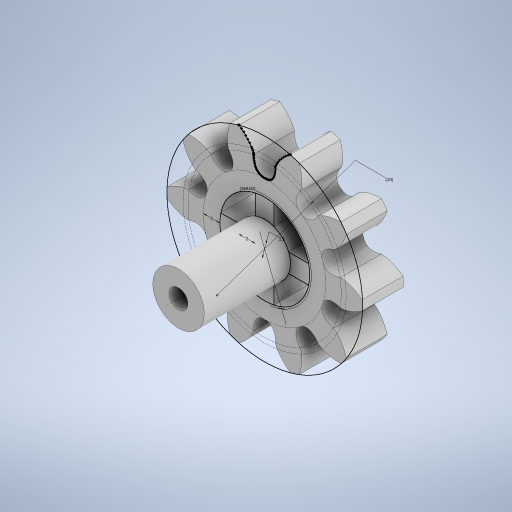
# Autodesk Inventor part: pinion_V3
Saved by Autodesk Inventor 2023 (Build 270158000, 158)
## iProperties
Created: 2022-11-24
Part Number: pinion_V3
Material: Generic
Document SubType Name: Modeling
Designer: shrey
Density: 1 g/cm^3
Appearance: Default
Author: shrey
Autodesk Inventor part; units mm, degrees
ref_plane "YZ Plane" through (0, 0, 0) normal (1, 0, 0) x (0, 1, 0)
ref_plane "XZ Plane" through (0, 0, 0) normal (0, 1, 0) x (-1, 0, 0)
ref_plane "XY Plane" through (0, 0, 0) normal (0, 0, 1) x (1, 0, 0)
sketch "Sketch1" plane through (0, 0, 0) normal (0, 0, 1) x (1, 0, 0)
  spline S0 degree 3 poles (-3.1449, 11.5806) (-3.0482, 11.5076) (-2.8549, 11.3615) (-2.5801, 11.1235) (-2.3181, 10.8715) (-2.0723, 10.6037) (-1.845, 10.3199) (-1.6746, 10.0692) (-1.5527, 9.8598) (-1.4703, 9.6979) (-1.3965, 9.5315) (-1.3613, 9.4156) (-1.3436, 9.3576) knots 0 0 0 0 0.125009 0.250018 0.375026 0.500029 0.625027 0.750014 0.81252 0.875024 0.937523 1 1 1 1
  spline S1 degree 3 poles (-1.3436, 9.3576) (-1.3456, 9.303) (-1.3494, 9.1938) (-1.3453, 9.0299) (-1.3323, 8.8664) (-1.3062, 8.7045) (-1.2743, 8.5436) (-1.2254, 8.3869) (-1.166, 8.2341) (-1.0913, 8.0878) (-1.0006, 7.951) (-0.8946, 7.8256) (-0.7725, 7.7154) (-0.6351, 7.6254) (-0.4861, 7.5557) (-0.3538, 7.5202) (-0.2459, 7.5023) (-0.1365, 7.4984) (0, 7.5011) (0.1365, 7.4984) (0.2459, 7.5023) (0.3538, 7.5202) (0.4861, 7.5557) (0.6351, 7.6254) (0.7725, 7.7154) (0.8946, 7.8256) (1.0006, 7.951) (1.0913, 8.0878) (1.166, 8.2341) (1.2254, 8.3869) (1.2743, 8.5436) (1.3062, 8.7045) (1.3323, 8.8664) (1.3453, 9.0299) (1.3494, 9.1938) (1.3456, 9.303) (1.3436, 9.3576) knots 0 0 0 0 0.016389 0.032777 0.049165 0.065552 0.081938 0.098325 0.114709 0.131097 0.147483 0.163864 0.180243 0.196616 0.21299 0.229355 0.237552 0.245745 0.262134 0.278522 0.286715 0.294912 0.311278 0.327651 0.344025 0.360403 0.376784 0.393171 0.409559 0.425942 0.44233 0.458716 0.475102 0.49149 0.507879 0.524268 0.524268 0.524268 0.524268
  spline S2 degree 3 poles (1.3436, 9.3576) (1.3613, 9.4156) (1.3965, 9.5315) (1.4703, 9.6979) (1.5527, 9.8598) (1.6746, 10.0692) (1.845, 10.3199) (2.0723, 10.6037) (2.3181, 10.8715) (2.5801, 11.1235) (2.8549, 11.3615) (3.0482, 11.5076) (3.1449, 11.5806) knots 0 0 0 0 0.062477 0.124976 0.18748 0.249986 0.374973 0.499971 0.624974 0.749982 0.874991 1 1 1 1
  circle A0 centre (0, 0) radius 7.5 construction
  circle A1 centre (0, 0) radius 9.3969 construction
  circle A2 centre (0, 0) radius 10 construction
  circle A3 centre (0, 0) radius 12
  circle A4 centre (0, 0) radius 1.15
  circle A5 centre (0, 0) radius 5.5
  circle A6 centre (0, 0) radius 3.15
  line L0 (-1.15, 2.9326) -> (-1.15, 5.3784)
  line L1 (1.15, 2.9326) -> (1.15, 5.3784)
  line L2 (-2.9326, -1.15) -> (-5.3784, -1.15)
  line L3 (-2.9326, 1.15) -> (-5.3784, 1.15)
  line L4 (1.15, -2.9326) -> (1.15, -5.3784)
  line L5 (-1.15, -2.9326) -> (-1.15, -5.3784)
  line L6 (2.9326, 1.15) -> (5.3784, 1.15)
  line L7 (2.9326, -1.15) -> (5.3784, -1.15)
  point P0 (-2.8575, 11.3584)
  point P1 (-2.5823, 11.1211)
  point P2 (-2.3208, 10.8689)
  point P3 (-2.0754, 10.601)
  point P4 (-1.8488, 10.317)
  point P5 (-1.6453, 10.0161)
  point P6 (-1.5542, 9.859)
  point P7 (-1.4717, 9.6971)
  point P8 (-1.4, 9.5302)
  point P9 (-1.3478, 9.1938)
  point P10 (-1.3438, 9.0299)
  point P11 (-1.3301, 8.8666)
  point P12 (-1.3053, 8.7047)
  point P13 (-1.2715, 8.5443)
  point P14 (-1.2237, 8.3876)
  point P15 (-1.1635, 8.2352)
  point P16 (-1.0887, 8.0894)
  point P17 (-0.998, 7.9529)
  point P18 (-0.8919, 7.8281)
  point P19 (-0.7699, 7.7188)
  point P20 (-0.6331, 7.6288)
  point P21 (-0.4845, 7.5602)
  point P22 (-0.3267, 7.5166)
  point P23 (-0.2457, 7.5041)
  point P24 (-0.1639, 7.4999)
  point P25 (0, 7.5)
  point P26 (0.1639, 7.4999)
  point P27 (0.2457, 7.5041)
  point P28 (0.3267, 7.5166)
  point P29 (0.4845, 7.5602)
  point P30 (0.6331, 7.6288)
  point P31 (0.7699, 7.7188)
  point P32 (0.8919, 7.8281)
  point P33 (0.998, 7.9529)
  point P34 (1.0887, 8.0894)
  point P35 (1.1635, 8.2352)
  point P36 (1.2237, 8.3876)
  point P37 (1.2715, 8.5443)
  point P38 (1.3053, 8.7047)
  point P39 (1.3301, 8.8666)
  point P40 (1.3438, 9.0299)
  point P41 (1.3478, 9.1938)
  point P42 (1.4, 9.5302)
  point P43 (1.4717, 9.6971)
  point P44 (1.5542, 9.859)
  point P45 (1.6453, 10.0161)
  point P46 (1.8488, 10.317)
  point P47 (2.0754, 10.601)
  point P48 (2.3208, 10.8689)
  point P49 (2.5823, 11.1211)
  point P50 (2.8575, 11.3584)
  point P51 (5.3784, -1.15)
  point P52 (2.9326, -1.15)
  point P53 (-1.15, -5.3784)
  point P54 (-2.9326, -1.15)
  point P55 (-5.3784, -1.15)
  point P56 (-5.3784, 1.15)
  point P57 (2.9326, 1.15)
  dimension "d2" = 2.3
  dimension "d3" = 2
  dimension "d4" = 2
  dimension "d7" = 360
  dimension "d18" = 20
  constraints: 16 end point, 7 centre point, 6 point on circle, 2 tangent, 1 coincident, 1 parallel, 1 vertical, 142 other
  measures "d2" diameter of A4
  measures "d3" radial gap between concentric circles of A0 A5
  measures "d4" radial gap between concentric circles of A4 A6
  measures "d18" diameter of A2
extrude "Extrusion1" add sketch "Sketch1" against normal blind 5 contours A3 S2 S1 S0 | S0 S1 S2 A3 | A4 | A5 L7 A6 L6 | L6 A6 L1 A5 | A5 L4 A6 L7 | L1 A6 L0 A5 | A6 | A5 L5 A6 L4 | L0 A6 L3 A5 | A5 L2 A6 L5 | L3 A6 L2 A5
extrude "Extrusion2" cut sketch "Sketch1" against normal through all contours A3 S2 S1 S0 picked at (0.367, 10.5472)
pattern_circular "Circular Pattern1" count 10 over 360 about axis through (0, 0, 0) along (0, 0, -1) of "Extrusion2"
extrude "Extrusion3" cut sketch "Sketch1" against normal through all contours A4 | L6 A6 L1 A5 | A5 L4 A6 L7 | L0 A6 L3 A5 | A5 L2 A6 L5
extrude "Extrusion4" add sketch "Sketch1" along normal blind 10.56 contours A6
equation "\"d0\" = FaceWidth"
equation "\"Module\" = 2"
equation "\"PressureAngle\" = 20deg"
equation "\"UnitProfileClearance\" = 0.25"
equation "\"UnitRoundRadius\" = 0.35"
equation "\"HeadDiameter\" = 24"
equation "\"RootDiameter\" = 15"
equation "\"BaseDiameter\" = 18.79385"
equation "\"FaceWidth\" = 5"
equation "\"HelixAngle\" = 0"
equation "\"UnitCorrection\" = 0"
equation "\"UnitAddendumModification\" = 0"
equation "\"CircularPitch\" = 6.283185"
equation "\"UnitBacklashShift\" = 0"
equation "\"TotalToolShift\" = 0"
equation "\"IsInternal\" = 0"
body "Solid1"
